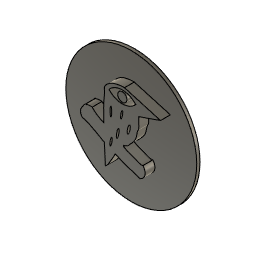
ring topper v8 (Autodesk Fusion 360 design; units mm, degrees)
Autodesk Fusion 360 part; units mm, degrees
note: some values were not read from the file. Set by a fixed rule: which sketch regions a step uses.
sketch "Sketch1" plane through (0, 0, 0) normal (0, 1, 0) x (1, 0, 0)
  circle A0 centre (0, 0) radius 10
  dimension "d1" = 20
  constraint coincident A0.centre origin
  measures "d1" diameter of A0
sketch "Sketch3" plane through (0, 0, 0) normal (0, 1, 0) x (1, 0, 0)
  circle A0 centre (-0.1315, -4.6672) radius 0.7107
  arc A1 (-2.1777, -4.689) -> (1.9146, -4.6672) centre (-0.1411, -2.8778) ccw
  arc A2 (1.9146, -4.6672) -> (-2.1777, -4.689) centre (-0.122, -6.4784) ccw
  line L0 (-5.9652, -4.4713) -> (-0.458, -6.0603)
  line L1 (-5.9652, -4.4713) -> (-2.6348, -3.3176)
  spline S0 degree 5 poles (-0.458, -6.0603) (-0.4244, -6.0611) (-0.3573, -6.0621) (-0.2577, -6.0621) (-0.1269, -6.0591) (0.0333, -6.0502) (0.1901, -6.0362) (0.3433, -6.0173) (0.4928, -5.9936) (0.6383, -5.9655) (0.7793, -5.9336) (0.9157, -5.8984) (1.0472, -5.8603) (1.1738, -5.8193) (1.2959, -5.7751) (1.4144, -5.7266) (1.5303, -5.6727) (1.6444, -5.6121) (1.7575, -5.5439) (1.8693, -5.4681) (1.9788, -5.3859) (2.0841, -5.2997) (2.1828, -5.2119) (2.2726, -5.1255) (2.3519, -5.0424) (2.4196, -4.964) (2.4759, -4.8903) (2.5213, -4.8205) (2.5568, -4.7539) (2.5834, -4.6894) (2.6016, -4.6264) (2.6097, -4.5771) (2.6123, -4.5406) (2.6124, -4.5166) (2.612, -4.5046) knots 0 0 0 0 0 0 0.033333 0.066667 0.1 0.133333 0.166667 0.2 0.233333 0.266667 0.3 0.333333 0.366667 0.4 0.433333 0.466667 0.5 0.533333 0.566667 0.6 0.633333 0.666667 0.7 0.733333 0.766667 0.8 0.833333 0.866667 0.9 0.933333 0.966667 1 1 1 1 1 1
  spline S1 degree 5 poles (5.4767, -0.9507) (5.4829, -0.9482) (5.4956, -0.9426) (5.5154, -0.9319) (5.543, -0.913) (5.5797, -0.882) (5.6182, -0.844) (5.6582, -0.7999) (5.6987, -0.7514) (5.7389, -0.7001) (5.7782, -0.6475) (5.816, -0.5943) (5.8525, -0.5405) (5.8884, -0.4851) (5.9242, -0.4271) (5.9607, -0.3664) (5.9982, -0.3035) (6.0364, -0.2406) (6.0748, -0.1797) (6.1124, -0.1223) (6.1482, -0.0681) (6.1805, -0.0146) (6.2079, 0.0423) (6.2291, 0.1062) (6.2435, 0.1792) (6.2513, 0.2599) (6.2536, 0.3434) (6.2518, 0.4237) (6.2472, 0.4956) (6.2407, 0.5559) (6.232, 0.6063) (6.2202, 0.6519) (6.2041, 0.6984) (6.1831, 0.7501) (6.1576, 0.8079) (6.1287, 0.8689) (6.0979, 0.9289) (6.0662, 0.9834) (6.0338, 1.0293) (5.9997, 1.0655) (5.9623, 1.0927) (5.9192, 1.1128) (5.8678, 1.1284) (5.8052, 1.1429) (5.7286, 1.1597) (5.6353, 1.1825) (5.5229, 1.2145) (5.3894, 1.2586) (5.233, 1.3171) (5.0525, 1.3918) (4.847, 1.4841) (4.6156, 1.5952) (4.3579, 1.7258) (4.0736, 1.8764) (3.7624, 2.0473) (3.4244, 2.2388) (3.1324, 2.4084) (2.9014, 2.5449) (2.742, 2.64) (2.6609, 2.6886) knots 0 0 0 0 0 0 0.018182 0.036364 0.054545 0.072727 0.090909 0.109091 0.127273 0.145455 0.163636 0.181818 0.2 0.218182 0.236364 0.254545 0.272727 0.290909 0.309091 0.327273 0.345455 0.363636 0.381818 0.4 0.418182 0.436364 0.454545 0.472727 0.490909 0.509091 0.527273 0.545455 0.563636 0.581818 0.6 0.618182 0.636364 0.654545 0.672727 0.690909 0.709091 0.727273 0.745455 0.763636 0.781818 0.8 0.818182 0.836364 0.854545 0.872727 0.890909 0.909091 0.927273 0.945455 0.963636 0.981818 1 1 1 1 1 1
  spline S2 degree 5 poles (2.612, -4.5046) (2.6087, -4.441) (2.6029, -4.3179) (2.5966, -4.1451) (2.5932, -3.9388) (2.5971, -3.7184) (2.6085, -3.5279) (2.6265, -3.3519) (2.649, -3.1634) (2.6732, -2.9341) (2.6959, -2.6428) (2.712, -2.2938) (2.7177, -1.9089) (2.7152, -1.4906) (2.7083, -1.0395) (2.7015, -0.5542) (2.6977, -0.0385) (2.6961, 0.4946) (2.6905, 1.017) (2.6793, 1.5085) (2.6628, 1.9537) (2.6428, 2.3435) (2.6219, 2.6753) (2.6025, 2.9534) (2.5857, 3.1903) (2.5713, 3.4051) (2.5585, 3.6195) (2.546, 3.8547) (2.5327, 4.1272) (2.5178, 4.4473) (2.5011, 4.821) (2.486, 5.165) (2.4737, 5.4487) (2.4651, 5.6493) (2.4607, 5.7524) knots 0 0 0 0 0 0 0.033333 0.066667 0.1 0.133333 0.166667 0.2 0.233333 0.266667 0.3 0.333333 0.366667 0.4 0.433333 0.466667 0.5 0.533333 0.566667 0.6 0.633333 0.666667 0.7 0.733333 0.766667 0.8 0.833333 0.866667 0.9 0.933333 0.966667 1 1 1 1 1 1
  line L2 (2.7038, -1.094) -> (2.6904, 1.435)
  line L3 (2.6446, -3.5336) -> (2.7495, -1.6246)
  spline S3 degree 5 poles (5.4767, -0.9507) (5.4709, -0.9483) (5.4591, -0.944) (5.4406, -0.9391) (5.4145, -0.9358) (5.379, -0.9371) (5.3404, -0.9436) (5.2983, -0.9549) (5.2516, -0.9699) (5.1994, -0.9871) (5.1403, -1.0047) (5.0731, -1.0208) (4.9969, -1.0339) (4.9111, -1.0426) (4.8156, -1.0465) (4.7106, -1.0454) (4.6191, -1.0404) (4.5465, -1.0344) (4.4962, -1.0294) (4.4706, -1.0267) knots 0 0 0 0 0 0 0.066667 0.133333 0.2 0.266667 0.333333 0.4 0.466667 0.533333 0.6 0.666667 0.733333 0.8 0.866667 0.933333 1 1 1 1 1 1
  spline S4 degree 5 poles (-3.2851, 2.8239) (-3.2636, 2.8326) (-3.2193, 2.8477) (-3.1488, 2.8631) (-3.0469, 2.8693) (-2.9063, 2.8537) (-2.7526, 2.8161) (-2.5859, 2.7596) (-2.4068, 2.689) (-2.2165, 2.6103) (-2.018, 2.5292) (-1.8159, 2.4509) (-1.6176, 2.3786) (-1.4311, 2.3138) (-1.2623, 2.2554) (-1.112, 2.2001) (-0.9732, 2.1418) (-0.8292, 2.0717) (-0.6597, 1.9806) (-0.4453, 1.8606) (-0.172, 1.7072) (0.163, 1.5208) (0.5519, 1.3074) (0.9797, 1.0759) (1.4267, 0.8372) (1.8709, 0.6029) (2.291, 0.3838) (2.6689, 0.1886) (2.9923, 0.0224) (3.2579, -0.1148) (3.4712, -0.2282) (3.6435, -0.326) (3.7886, -0.4177) (3.9205, -0.5125) (4.0497, -0.6173) (4.1824, -0.7362) (4.2939, -0.8441) (4.3809, -0.9325) (4.4405, -0.9947) (4.4706, -1.0267) knots 0 0 0 0 0 0 0.028571 0.057143 0.085714 0.114286 0.142857 0.171429 0.2 0.228571 0.257143 0.285714 0.314286 0.342857 0.371429 0.4 0.428571 0.457143 0.485714 0.514286 0.542857 0.571429 0.6 0.628571 0.657143 0.685714 0.714286 0.742857 0.771429 0.8 0.828571 0.857143 0.885714 0.914286 0.942857 0.971429 1 1 1 1 1 1
  arc A3 (-2.816, 4.7931) -> (-3.2851, 2.8239) centre (-2.4277, 3.6601) ccw
  spline S5 degree 5 poles (-2.816, 4.7931) (-2.7857, 4.7796) (-2.7248, 4.7528) (-2.6323, 4.7138) (-2.5068, 4.6638) (-2.3462, 4.6048) (-2.1826, 4.5493) (-2.0169, 4.4969) (-1.8509, 4.4472) (-1.6869, 4.3997) (-1.5272, 4.3536) (-1.3733, 4.3078) (-1.2251, 4.2614) (-1.0799, 4.2132) (-0.9332, 4.162) (-0.7804, 4.1069) (-0.6182, 4.0477) (-0.4462, 3.9845) (-0.2681, 3.9187) (-0.0897, 3.8518) (0.0827, 3.7853) (0.2447, 3.7203) (0.3954, 3.6568) (0.5388, 3.5935) (0.6823, 3.528) (0.8347, 3.4579) (1.0047, 3.3806) (1.1994, 3.294) (1.4233, 3.1969) (1.6794, 3.0884) (1.9692, 2.9681) (2.2286, 2.8623) (2.4387, 2.7775) (2.5857, 2.7186) (2.6609, 2.6886) knots 0 0 0 0 0 0 0.033333 0.066667 0.1 0.133333 0.166667 0.2 0.233333 0.266667 0.3 0.333333 0.366667 0.4 0.433333 0.466667 0.5 0.533333 0.566667 0.6 0.633333 0.666667 0.7 0.733333 0.766667 0.8 0.833333 0.866667 0.9 0.933333 0.966667 1 1 1 1 1 1
  spline S6 degree 5 poles (2.4607, 5.7524) (2.4295, 5.724) (2.3695, 5.6688) (2.2867, 5.5906) (2.191, 5.4955) (2.095, 5.3914) (2.0209, 5.3001) (1.9644, 5.2179) (1.9186, 5.1381) (1.8733, 5.0513) (1.818, 4.9475) (1.7444, 4.8182) (1.6483, 4.6585) (1.5323, 4.4686) (1.4026, 4.253) (1.2675, 4.0192) (1.1359, 3.7774) (1.0144, 3.5392) (0.9065, 3.3173) (0.8098, 3.1243) (0.7183, 2.971) (0.625, 2.8646) (0.5236, 2.8069) (0.4107, 2.7924) (0.2883, 2.8061) (0.1623, 2.8268) (0.0402, 2.8313) (-0.0701, 2.7977) (-0.1629, 2.71) (-0.2346, 2.5582) (-0.283, 2.3364) (-0.3025, 2.101) (-0.3061, 1.8916) (-0.3036, 1.7374) (-0.3012, 1.6566) knots 0 0 0 0 0 0 0.033333 0.066667 0.1 0.133333 0.166667 0.2 0.233333 0.266667 0.3 0.333333 0.366667 0.4 0.433333 0.466667 0.5 0.533333 0.566667 0.6 0.633333 0.666667 0.7 0.733333 0.766667 0.8 0.833333 0.866667 0.9 0.933333 0.966667 1 1 1 1 1 1
  spline S7 degree 5 poles (-2.6348, -3.3176) (-2.636, -3.2414) (-2.6384, -3.0925) (-2.6419, -2.8801) (-2.6465, -2.6186) (-2.6515, -2.3285) (-2.6547, -2.0759) (-2.653, -1.8633) (-2.6428, -1.6916) (-2.615, -1.568) (-2.5661, -1.4884) (-2.5109, -1.4184) (-2.4649, -1.3217) (-2.4272, -1.1821) (-2.3874, -1.0056) (-2.3447, -0.7977) (-2.2962, -0.5689) (-2.2388, -0.3304) (-2.1601, -0.0928) (-2.0452, 0.1355) (-1.9001, 0.3481) (-1.7379, 0.541) (-1.5769, 0.712) (-1.4334, 0.8607) (-1.317, 0.9884) (-1.2249, 1.0981) (-1.1467, 1.1938) (-1.0681, 1.2797) (-0.9747, 1.3595) (-0.8564, 1.436) (-0.7077, 1.5106) (-0.5621, 1.5694) (-0.4375, 1.6132) (-0.3478, 1.6422) (-0.3012, 1.6566) knots 0 0 0 0 0 0 0.033333 0.066667 0.1 0.133333 0.166667 0.2 0.233333 0.266667 0.3 0.333333 0.366667 0.4 0.433333 0.466667 0.5 0.533333 0.566667 0.6 0.633333 0.666667 0.7 0.733333 0.766667 0.8 0.833333 0.866667 0.9 0.933333 0.966667 1 1 1 1 1 1
  line L4 (-2.7052, -2.115) -> (-2.5644, -1.2422)
  line L5 (-2.6348, -1.782) -> (-2.299, -0.8403)
  line L6 (-2.4311, -0.9624) -> (-2.0065, 0.3983)
  ellipse E0 centre (-1.1127, -0.8458) end of major axis (-1.2771, -1.5361) minor radius 0.1766
  line L7 (-0.9483, -0.1555) -> (-1.2771, -1.5361)
  line L8 (-1.2845, -0.8049) -> (-0.9409, -0.8867)
  ellipse E1 centre (-0.0279, -2.2593) end of major axis (-0.1411, -2.8778) minor radius 0.1263
  line L9 (0.0853, -1.6408) -> (-0.1411, -2.8778)
  line L10 (-0.1521, -2.2366) -> (0.0963, -2.282)
  ellipse E2 centre (1.6157, -1.8648) end of major axis (1.6157, -2.588) minor radius 0.1224
  line L11 (1.6157, -1.1416) -> (1.6157, -2.588)
  line L12 (1.4933, -1.8648) -> (1.7381, -1.8648)
  ellipse E3 centre (0.5638, 0.492) end of major axis (0.7064, 1.2242) minor radius 0.1533
  line L13 (0.4212, -0.2402) -> (0.7064, 1.2242)
  line L14 (0.7142, 0.4627) -> (0.4134, 0.5213)
  ellipse E4 centre (1.5993, 2.1127) end of major axis (1.476, 1.4797) minor radius 0.1314
  line L15 (1.7226, 2.7457) -> (1.476, 1.4797)
  line L16 (1.4703, 2.1379) -> (1.7282, 2.0876)
  point P0 (0.4556, -5.9987)
  point P1 (1.1908, -5.8122)
  point P2 (1.7932, -5.5185)
  point P3 (2.3119, -5.0834)
  point P4 (2.5541, -4.7554)
  point P5 (5.6115, -0.8498)
  point P6 (5.7831, -0.6401)
  point P7 (5.9451, -0.3923)
  point P8 (6.1166, -0.1159)
  point P9 (6.2358, 0.1451)
  point P10 (6.2453, 0.5084)
  point P11 (6.1977, 0.7133)
  point P12 (6.0785, 0.9611)
  point P13 (5.9356, 1.104)
  point P14 (5.6074, 1.1911)
  point P15 (2.612, -3.5085)
  point P16 (2.6971, -2.5791)
  point P17 (2.6971, 0.1705)
  point P18 (2.612, 2.8146)
  point P19 (2.5514, 3.7569)
  point P20 (5.3154, -0.9507)
  point P21 (5.0352, -1.0267)
  point P22 (-2.7943, 2.8239)
  point P23 (-1.9668, 2.51)
  point P24 (-1.1507, 2.2133)
  point P25 (-0.3517, 1.8081)
  point P26 (2.8271, 0.1074)
  point P27 (3.8658, -0.4747)
  point P28 (-2.0661, 4.5129)
  point P29 (-1.3209, 4.2911)
  point P30 (-0.6289, 4.0515)
  point P31 (0.214, 3.7321)
  point P32 (0.9149, 3.4216)
  point P33 (1.9844, 5.245)
  point P34 (1.7529, 4.8347)
  point P35 (1.0164, 3.5405)
  point P36 (0.5113, 2.8146)
  point P37 (0.0063, 2.8146)
  point P38 (-2.6348, -1.6786)
  point P39 (-2.4669, -1.3111)
  point P40 (-2.2188, -0.282)
  point P41 (-1.447, 0.8481)
  point P42 (-1.0427, 1.2983)
  constraint midpoint P17 L2
  constraint midpoint P16 L3
  constraint midpoint P38 L4
  constraint midpoint P39 L5
  constraint midpoint P40 L6
  constraint coincident E0 L7.start
  constraint coincident E0 L7.end
  constraint coincident E0 L8.start
  constraint coincident E0 L8.end
  constraint coincident E1 L9.start
  constraint coincident A1.centre E1
  constraint coincident E1 L10.start
  constraint coincident E1 L10.end
  constraint coincident E2 L11.start
  constraint coincident E2 L11.end
  constraint coincident E2 L12.start
  constraint coincident E2 L12.end
  constraint vertical L11
  constraint coincident E3 L13.start
  constraint coincident E3 L13.end
  constraint coincident E3 L14.start
  constraint coincident E3 L14.end
  constraint coincident E4 L15.start
  constraint coincident E4 L15.end
  constraint coincident E4 L16.start
  constraint coincident E4 L16.end
  constraint parallel L13 L15
extrude "Extrude1" add sketch "Sketch1" along normal blind 2 makes body 1
extrude "Extrude2" cut sketch "Sketch3" along normal blind 1.5 contours L0 L1 S0 S2 L2 S4 S6 S7 | S2 S4 S5 S6 | S2 S5 S6 bodies 1
extrude "Extrude3" cut sketch "Sketch3" along normal blind 1 contours S1 S2 S3 S4 S5 | S4 A3 S5 S6 bodies 1
extrude "Extrude4" cut sketch "Sketch3" along normal blind 1.5 contours A0 bodies 1
move_body "Move1" bodies 1 to x (1, 0, 0) y (0, 1, 0) z (0, 0, 1) at (-20, 0, 0)
extrude "Extrude5" add sketch "Sketch1" along normal blind 2 separate body makes body 2
move_face "MoveFace1" to x (1, 0, 0) y (0, 1, 0) z (0, 0, 1) at (0, -6, 0) 1 faces at (9.9876, 1.3333, 0.4985) on bodies 2
move_face "MoveFace2" to x (1, 0, 0) y (0, 1, 0) z (0, 0, 1) at (0, -4, 0) 1 faces at (9.9876, 1.3333, 0.4985) on bodies 2
move_face "MoveFace3" to x (1, 0, 0) y (0, 1, 0) z (0, 0, 1) at (0, -13, 0) 1 faces at (9.9876, 1.3333, 0.4985) on bodies 2
move_body "Move2" bodies 2 to x (1, 0, 0) y (0, 1, 0) z (0, 0, 1) at (3, 2, 0)
move_face "MoveFace4" by (20, 0, 0) 1 faces at (-25.2154, 0, -0.6489) on bodies 1
move_body "Move3" bodies 2 to x (1, 0, 0) y (0, 1, 0) z (0, 0, 1) at (0, -4, 0)
move_body "Move4" bodies 1 to x (1, 0, 0) y (0, 1, 0) z (0, 0, 1) at (23, 0, 0)
extrude "Extrude6" cut 7 faces at (-2.2154, 0, -0.6489) (1.657, 0, 4.6796) (2.9067, 0, 2.4067) (1.7929, 0, 1.012) (3.6449, 0, -0.6679) (4.6511, 0, 1.9852) (4.6688, 0, -2.2639) along direction (0, -1, 0) blind 1.5 on bodies 1 bodies 2
move_body "Move5" bodies 2 to x (1, 0, 0) y (0, 1, 0) z (0, 0, 1) at (-2.5114, 1.9963, 10.02)
move_body "Move6" bodies 2 to x (-1, 0, 0) y (0, -1, 0) z (0, 0, 1) at (0.9772, -0.0073, 0)
hidden bodies 1
